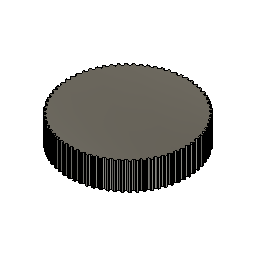
gear_70z (Autodesk Fusion 360 design; units mm, degrees)
Autodesk Fusion 360 part; units mm, degrees
sketch "Sketch1" plane through (0, 0, 0) normal (0, 0, 1) x (1, 0, 0) in component "gt2 pulley"
  circle A0 centre (0, 0) radius 22.2817 construction
  circle A1 centre (0, 0) radius 21.2777 construction
  line L0 (0, 0) -> (0, 22.2817) construction
  line L1 (0, 0) -> (0.9997, 22.2593) construction
  line L2 (0, 0) -> (1.4055, 22.2373) construction
  circle A2 centre (0, 0) radius 22.0277 construction
  arc A3 (0.3938, 21.8903) -> (0.4682, 21.5948) centre (1.3895, 21.9838) ccw
  circle A4 centre (0, 0) radius 21.8777 construction
  arc A5 (0.2461, 22.0263) -> (0, 22.0277) centre (0, 0) ccw
  arc A6 (0.3938, 21.8903) -> (0.2461, 22.0263) centre (0.2445, 21.8763) ccw
  arc A7 (0.4682, 21.5948) -> (0.9546, 21.2563) centre (0.9795, 21.8107) ccw
  arc A8 (0, 22.0277) -> (-0.2461, 22.0263) centre (0, 0) ccw
  arc A9 (-0.2461, 22.0263) -> (-0.3938, 21.8903) centre (-0.2445, 21.8763) ccw
  arc A10 (-0.4682, 21.5948) -> (-0.3938, 21.8903) centre (-1.3895, 21.9838) ccw
  arc A11 (-0.9545, 21.2563) -> (-0.4682, 21.5948) centre (-0.9795, 21.8107) ccw
  arc A12 (0.9546, 21.2563) -> (-0.9546, 21.2563) centre (0, 0) ccw
  point P0 (1.3895, 21.9838)
  point P1 (0, 22.0277)
  dimension "d18" = 44.5634
  dimension "d19" = 2.571
  dimension "d22" = 1.004
  dimension "d24" = 0.75
  dimension "d26" = 1
  dimension "d27" = 0.15
  dimension "d28" = 0.15
  dimension "d47" = 0.555
  dimension "d52" = 3.812
  constraint coincident A0.centre A1.centre
  constraint coincident A0 L0.end
  constraint vertical L0
  constraint coincident A0 L1.end
  constraint coincident A0 L2.end
  constraint concentric A1 A2
  constraint coincident A1 A7.end
  constraint coincident L1 A7.end
  constraint coincident A2 P0
  constraint coincident L2 P0
  constraint coincident P0 A3.centre
  constraint coincident A2 P1
  constraint coincident L0 P1
  constraint concentric A2 A4
  constraint coincident P1 A5.end
  constraint coincident A4 A6.centre
  constraint coincident A3.start A6.start
  constraint tangent A3 A6
  constraint tangent A3 A7
  constraint symmetric L0 A7.end A12.end
  constraint symmetric L0 A3.start A9.end
  constraint symmetric L0 A3.end A10.start
  constraint symmetric L0 A3 A10
  constraint symmetric L0 A5.start A8.end
  constraint symmetric L0 P1 A5.end
  constraint symmetric L0 A5 A8
  constraint symmetric L0 A6 A9
  constraint symmetric L0 A7 A11
  constraint coincident A1 A11.start
  constraint tangent A1 A7
  constraint coincident L1 A7.centre
  measures "d18" diameter of A0
  measures "d19" angle of L0 L1
  measures "d22" distance of A0 A1
  measures "d24" distance of A1 A2
  measures "d26" radius of A3
  measures "d27" distance of A2 A4
  measures "d28" radius of A6
  measures "d47" radius of A7
extrude "Extrude1" add sketch "Sketch1" along normal blind 10 makes body 1
pattern_circular "C-Pattern1" count 70 over 360 about axis through (0, 0, 1.75) along (0, 0, 1) of bodies 1 makes body 2 at (-1.1666, 21.2457, 3.3333) makes body 3 at (-4.5275, 20.7904, 6.6667) makes body 4 at (-6.1702, 20.3634, 6.6667) makes body 5 at (-6.7767, 20.1697, 3.3333) makes body 6 at (-8.5574, 19.4811, 3.3333) makes body 7 at (-11.5441, 17.8739, 6.6667) makes body 8 at (-13.0998, 16.7671, 6.6667) makes body 9 at (-14.3945, 15.6697, 6.6667) makes body 10 at (-14.8569, 15.232, 3.3333) makes body 11 at (-16.1624, 13.8389, 3.3333) makes body 12 at (-18.156, 11.095, 6.6667) makes body 13 at (-19.0775, 9.4228, 6.6667) makes body 14 at (-19.8453, 7.6748, 6.6667) makes body 15 at (-19.9945, 7.2774, 3.3333) makes body 16 at (-20.5663, 5.4558, 3.3333) makes body 17 at (-21.1498, 2.3297, 6.6667) makes body 18 at (-21.21, 1.6959, 3.3333) makes body 19 at (-21.21, -1.6958, 6.6667) makes body 20 at (-21.0991, -2.751, 6.6667) makes body 21 at (-20.6197, -5.2504, 6.6667) makes body 22 at (-19.9945, -7.2773, 6.6667) makes body 23 at (-19.8454, -7.6747, 3.3333) makes body 24 at (-18.6866, -10.1761, 6.6667) makes body 25 at (-18.1561, -11.0949, 3.3333) makes body 26 at (-16.1625, -13.8389, 6.6667) makes body 27 at (-15.3059, -14.7807, 6.6667) makes body 28 at (-13.5956, -16.3676, 6.6667) makes body 29 at (-12.4208, -17.2761, 6.6667) makes body 30 at (-10.8221, -18.32, 6.6667) makes body 31 at (-9.1364, -19.2163, 6.6667) makes body 32 at (-8.1671, -19.6479, 3.3333) makes body 33 at (-6.373, -20.3009, 3.3333) makes body 34 at (-3.0664, -21.0556, 6.6667) makes body 35 at (-2.6458, -21.1126, 3.3333) makes body 36 at (0.7425, -21.2647, 6.6667) makes body 37 at (2.0129, -21.1823, 6.6667) makes body 38 at (4.5275, -20.7904, 6.6667) makes body 39 at (6.1702, -20.3634, 6.6667) makes body 40 at (6.7767, -20.1697, 3.3333) makes body 41 at (8.5574, -19.4811, 3.3333) makes body 42 at (11.5441, -17.8739, 6.6667) makes body 43 at (13.0998, -16.7671, 6.6667) makes body 44 at (14.0791, -15.9536, 6.6667) makes body 45 at (14.8569, -15.232, 3.3333) makes body 46 at (17.0884, -12.6778, 6.6667) makes body 47 at (18.156, -11.095, 6.6667) makes body 48 at (18.7871, -9.9893, 6.6667) makes body 49 at (19.8453, -7.6748, 6.6667) makes body 50 at (19.9945, -7.2774, 3.3333) makes body 51 at (20.5663, -5.4558, 3.3333) makes body 52 at (21.1498, -2.3297, 6.6667) makes body 53 at (21.21, -1.6959, 3.3333) makes body 54 at (21.21, 1.6958, 6.6667) makes body 55 at (21.0991, 2.751, 6.6667) makes body 56 at (20.6197, 5.2504, 6.6667) makes body 57 at (20.2033, 6.676, 6.6667) makes body 58 at (19.8454, 7.6747, 3.3333) makes body 59 at (18.3738, 10.7305, 6.6667) makes body 60 at (17.3379, 12.3344, 6.6667) makes body 61 at (16.1625, 13.8389, 6.6667) makes body 62 at (15.8832, 14.1585, 3.3333) makes body 63 at (13.5956, 16.3676, 6.6667) makes body 64 at (11.8984, 17.64, 6.6667) makes body 65 at (11.5441, 17.8738, 3.3333) makes body 66 at (9.8955, 18.8367, 3.3333) makes body 67 at (8.1671, 19.6479, 3.3333) makes body 68 at (5.5583, 20.5389, 6.6667) makes body 69 at (3.0664, 21.0556, 6.6667) makes body 70 at (1.1666, 21.2457, 6.6667)
sketch "Sketch2" plane through (0, 0, 10) normal (0, 0, 1) x (-1, 0, 0)
  arc A0 (-9.8527, -19.5516) -> (-9.7786, -19.7382) centre (-9.7121, -19.6038) ccw
  arc A1 (-9.7786, -19.7382) -> (-9.3351, -19.9518) centre (0, 0) ccw
  arc A2 (-9.3351, -19.9518) -> (-9.143, -19.8934) centre (-9.2715, -19.816) ccw
  arc A3 (-8.9478, -19.6594) -> (-9.143, -19.8934) centre (-8.2866, -20.4096) ccw
  arc A4 (-8.3627, -19.5654) -> (-8.9478, -19.6594) centre (-8.5808, -20.0758) ccw
  arc A5 (-10.0828, -18.737) -> (-8.3627, -19.5654) centre (0, 0) ccw
  arc A6 (-9.7915, -19.2531) -> (-10.0828, -18.737) centre (-10.3458, -19.2258) ccw
  arc A7 (-9.8527, -19.5516) -> (-9.7915, -19.2531) centre (-10.7903, -19.2039) ccw
  circle A8 centre (0, 0) radius 21.2777
  constraint coincident A1.centre A5.centre
extrude "Extrude2" add sketch "Sketch2" against normal blind 10 contours A5 A8 bodies 1 2 3 4 5 6 7 8 9 10 11 12 13 14 15 16 17 18 19 20 21 22 23 24 25 26 27 28 29 30 31 32 33 34 35 36 37 38 39 40 41 42 43 44 45 46 47 48 49 50 51 52 53 54 55 56 57 58 59 60 61 62 63 64 65 66 67 68 69 70
extrude "Extrude4" [suppressed] in component "gt2 pulley"
pattern_circular "C-Pattern7" [suppressed] in component "gt2 pulley"
extrude "Extrude3" [suppressed] in component "gt2 pulley"
pattern_circular "C-Pattern6" [suppressed] in component "gt2 pulley"
extrude "Extrude2'" [suppressed] in component "gt2 pulley"
pattern_circular "C-Pattern5" [suppressed] in component "gt2 pulley"
extrude "Extrude1'" [suppressed] in component "gt2 pulley"
pattern_circular "C-Pattern4" [suppressed] in component "gt2 pulley"
pattern_circular "C-Pattern3" [suppressed] in component "gt2 pulley"
pattern_circular "C-Pattern2" [suppressed] in component "gt2 pulley"
pattern_circular "C-Pattern1'" [suppressed] in component "gt2 pulley"
copy_body "Body->Comp1" [suppressed] in component "Component"
copy_body "Body->Comp2" [suppressed] in component "Component'"
copy_body "Body->Comp3" [suppressed] in component "Component''"
copy_body "Body->Comp4" [suppressed] in component "Component'''"
copy_body "Body->Comp5" [suppressed] in component "Component''''"
copy_body "Body->Comp6" [suppressed] in component "Component'''''"
copy_body "Body->Comp7" [suppressed] in component "Component''''''"
copy_body "Body->Comp8" [suppressed] in component "Component'''''''"
copy_body "Body->Comp9" [suppressed] in component "Component''''''''"
copy_body "Body->Comp10" [suppressed] in component "Component'''''''''"
copy_body "Body->Comp11" [suppressed] in component "Component''''''''''"
copy_body "Body->Comp12" [suppressed] in component "Component'''''''''''"
copy_body "Body->Comp13" [suppressed] in component "Component''''''''''''"
copy_body "Body->Comp14" [suppressed] in component "Component'''''''''''''"
copy_body "Body->Comp15" [suppressed] in component "Component''''''''''''''"
copy_body "Body->Comp16" [suppressed] in component "Component'''''''''''''''"
copy_body "Body->Comp17" [suppressed] in component "Component''''''''''''''''"
copy_body "Body->Comp18" [suppressed] in component "Component'''''''''''''''''"
copy_body "Body->Comp19" [suppressed] in component "Component''''''''''''''''''"
copy_body "Body->Comp20" [suppressed] in component "Component'''''''''''''''''''"
component "gt2 pulley" placed x (1, 0, 0) y (0, 1, 0) z (0, 0, 1) at (0, 0, 0)
equation "NumTeeth = 70" comment "min 20"
equation "ToothPitch = 2 mm"
equation "PullyDia = NumTeeth * ToothPitch / PI"
equation "ToothAng = ( ( 360 / NumTeeth ) * 1 deg )"
equation "TransOffsetAngle = ToothAng * 0.2"
equation "Sholulder_Radius = 0.15 mm"
equation "Root_Radius = 0.555 mm"
equation "TransRadius = 1 mm"
equation "ToolHeight = 0.75 mm"
equation "PLD = 0.254 mm"
equation "d18 = PullyDia"
equation "d19 = ToothAng / 2"
equation "d22 = PLD + ToolHeight"
equation "d24 = ToolHeight"
equation "d26 = TransRadius"
equation "d27 = Sholulder_Radius"
equation "d31 = NumTeeth"
equation "d33 = NumTeeth"
equation "d35 = NumTeeth"
equation "d37 = NumTeeth"
equation "d41 = NumTeeth"
equation "d45 = NumTeeth"
equation "d47 = Root_Radius"
equation "d50 = NumTeeth"
